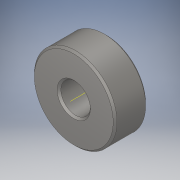
# Autodesk Inventor part: R10-2RS Ball Bearing 5_8x1-3_8x11_32 Sealed S7PP 99R10
Saved by Autodesk Inventor 2019.4 (Build 234330000, 330)
## iProperties
Created: 2018-01-08
Part Number: R10-2RS Ball Bearing 5_8x1-3_8x11_32 Sealed S7PP 99R10
Material: Steel
Document SubType Name: Modeling
Designer: dlangdon
Density: 7.85 g/cm^3
Appearance: Stainless - Brushed
Mass: 12.7982 g
Surface Area: 9.64933 cm^2
Volume: 1.63034 cm^3
Author: dlangdon
Autodesk Inventor part; units mm, degrees
ref_plane "YZ Plane" through (0, 0, 0) normal (1, 0, 0) x (0, 1, 0)
ref_plane "XZ Plane" through (0, 0, 0) normal (0, 1, 0) x (-1, 0, 0)
ref_plane "XY Plane" through (0, 0, 0) normal (0, 0, 1) x (1, 0, 0)
sketch "Sketch1" plane through (0, 0, 0) normal (0, 0, 1) x (1, 0, 0)
  circle A0 centre (0, 0) radius 3.9688
  circle A1 centre (0, 0) radius 11.1125
  dimension "d7" = 7.9375
  dimension "d8" = 22.225
  constraints: 2 centre point, 2 coincident
  measures "d7" diameter of A0
  measures "d8" diameter of A1
extrude "Extrusion1" add sketch "Sketch1" along normal blind 8.7313
chamfer "Chamfer1" distance 0.508 angle 45 4 edges at (-11.1125, 0, 8.7313) (-3.9688, 0, 8.7313) (-3.9688, 0, 0) (-11.1125, 0, 0)
ref_plane "Work Plane1" through (0, 0, 4.3656) normal (0, 0, 1) x (1, 0, 0)
ref_plane "Work Plane2" through (0, 0, 4.3656) normal (0, 0, 1) x (1, 0, 0)
body "Solid1"
